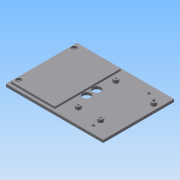
# Autodesk Inventor part: base_plate_r2
Saved by Autodesk Inventor 2014 (Build 180170000, 170)
## iProperties
Created: 2014-07-01
Part Number: base_plate_r2
Material: Generic
Document SubType Name: Modeling
Designer: Workstation
Density: 1 g/cm^3
Appearance: Default
Author: Workstation
Autodesk Inventor part; units mm, degrees
ref_plane "YZ Plane" through (0, 0, 0) normal (1, 0, 0) x (0, 1, 0)
ref_plane "XZ Plane" through (0, 0, 0) normal (0, 1, 0) x (-1, 0, 0)
ref_plane "XY Plane" through (0, 0, 0) normal (0, 0, 1) x (1, 0, 0)
sketch "Sketch1" plane through (0, 0, 0) normal (0, 1, 0) x (-1, 0, 0)
  line L0 (-16.8496, 81.8638) -> (105.0704, 81.8638)
  line L1 (105.0704, 81.8638) -> (105.0704, -7.0362)
  line L2 (105.0704, -7.0362) -> (-16.8496, -7.0362)
  line L3 (-16.8496, -7.0362) -> (-16.8496, 81.8638)
  point P0 (0, 0)
  dimension "d0" = 121.92
  dimension "d1" = 88.9
  constraints: 8 end point, 2 parallel, 1 horizontal, 1 perpendicular
  measures "d0" distance of L1.end L2.end
  measures "d1" distance of L0.end L1.end
extrude "Extrusion1" add sketch "Sketch1" along normal blind 3.429
sketch "Sketch2" plane through (0, 3.429, 0) normal (0, 1, 0) x (1, 0, 0)
  line L0 (-105.0704, -81.8638) -> (16.8496, -81.8638) projected
  line L1 (16.8496, 7.0362) -> (-105.0704, 7.0362) projected
  line L2 (-105.0704, 7.0362) -> (-105.0704, -81.8638) projected
  circle A0 centre (-98.7204, -2.6158) radius 1.5875
  circle A1 centre (-98.7204, -72.2118) radius 1.5875
  circle A2 centre (-4.7404, -2.6158) radius 1.5875
  circle A3 centre (-4.7404, -72.2118) radius 1.5875
  point P0 (0, 0)
  dimension "d4" = 121.92
  dimension "d5" = 88.9
  dimension "d6" = 6.35
  dimension "d8" = 6.35
  dimension "d12" = 3.175
  dimension "d13" = 3.175
  dimension "d15" = 3.175
  dimension "d18" = 93.98
  dimension "d20" = 69.596
  dimension "d21" = 9.652
  dimension "d22" = 9.652
  dimension "d23" = 3.175
  dimension "d64" = 9.652
  dimension "d65" = 9.652
  constraints: 4 centre point, 4 coincident
  measures "d4" distance of L0.start L0.end
  measures "d5" distance of L0.end L1.start
  measures "d6" distance from line of point (-98.72, -2.616) L2
  measures "d8" distance from line of point (-98.72, -72.212) L2
  measures "d12" diameter of A0
  measures "d13" diameter of A1
  measures "d15" diameter of A2
  measures "d18" distance of A0.centre A2.centre
  measures "d20" distance of A1.centre A0.centre
  measures "d21" distance from line of L1 A0.centre
  measures "d22" distance from line of L0 A1.centre
  measures "d23" diameter of A3
  measures "d64" distance from line of L1 A2.centre
  measures "d65" distance from line of L0 A3.centre
extrude "Extrusion3" cut sketch "Sketch2" against normal through all
sketch "Sketch4" plane through (0, 3.429, 0) normal (0, 1, 0) x (1, 0, 0)
  circle A0 centre (-98.7204, -2.6158) radius 1.5875 projected
  circle A1 centre (-98.7204, -72.2118) radius 1.5875 projected
  line L0 (16.8496, 7.0362) -> (-105.0704, 7.0362) projected
  line L1 (-105.0704, 7.0362) -> (-105.0704, -81.8638) projected
  line L2 (-101.8954, -78.6888) -> (-47.0314, -78.6888)
  line L3 (-47.0314, -78.6888) -> (-47.0314, 3.8612)
  line L4 (-47.0314, 3.8612) -> (-101.8954, 3.8612)
  line L5 (-101.8954, 3.8612) -> (-101.8954, -78.6888)
  circle A2 centre (-98.7204, -2.6158) radius 3.175
  circle A3 centre (-98.7204, -72.2118) radius 3.175
  point P0 (0, 0)
  dimension "d26" = 54.864
  dimension "d27" = 82.55
  dimension "d28" = 3.175
  dimension "d29" = 3.175
  dimension "d38" = 3.175
  constraints: 8 end point, 2 centre point, 2 coincident, 2 parallel, 2 perpendicular, 2 tangent
  measures "d26" distance of L2.start L2.end
  measures "d27" distance of L2.end L3.end
  measures "d28" distance between parallel lines of L4 L0
  measures "d29" distance between parallel lines of L5 L1
  measures "d38" distance from line of L5 A2.centre
extrude "Extrusion4" add sketch "Sketch4" along normal blind 2.54 contours L5 L4 L3 L2
sketch "Sketch5" plane through (0, 3.429, 0) normal (0, 1, 0) x (1, 0, 0)
  line L0 (-47.0314, 3.8612) -> (-47.0314, -78.6888) projected
  line L1 (-47.0314, -37.4138) -> (-47.0314, -31.0638)
  line L2 (-47.0314, -31.0638) -> (-47.0314, -43.7638)
  line L3 (-47.0314, -43.7638) -> (-41.9514, -43.7638)
  circle A0 centre (-41.9514, -43.7638) radius 5.08
  circle A1 centre (-41.9514, -31.0638) radius 5.08
  point P0 (0, 0)
  dimension "d35" = 6.35
  dimension "d36" = 12.7
  dimension "d37" = 5.08
  constraints: 6 end point, 2 horizontal alignment, 2 point on line, 1 coincident, 1 midpoint, 1 perpendicular, 4 other
  measures "d35" distance of L1.start L1.end
  measures "d36" distance of L1.end L2.end
  measures "d37" distance of L2.end L3.end
extrude "Extrusion5" cut sketch "Sketch5" against normal through all
sketch "Sketch6" plane through (0, 3.429, 0) normal (0, 1, 0) x (1, 0, 0)
  line L0 (-47.0314, -31.0638) -> (-47.0314, -43.7638) projected
  line L1 (-105.0704, 7.0362) -> (-105.0704, -81.8638) projected
  line L2 (-47.0314, -37.4138) -> (-40.6814, -37.4138)
  line L3 (-40.6814, -37.4138) -> (-40.6814, -65.3538)
  line L4 (-40.6814, -65.3538) -> (-40.6814, 3.1754)
  line L5 (-40.6814, 3.1754) -> (12.6586, 3.1754)
  line L6 (12.6586, 3.1754) -> (12.6586, -65.3538)
  line L7 (12.6586, -65.3538) -> (-40.6814, -65.3538)
  line L8 (-40.6814, -65.3538) -> (-40.6814, -63.0678)
  line L9 (-40.6814, -63.0678) -> (12.6586, -63.0678)
  line L10 (-40.6814, -63.0678) -> (-33.0614, -63.0678)
  line L11 (-33.0614, -63.0678) -> (-5.1214, -63.0678)
  circle A0 centre (-33.0614, -63.0678) radius 3.175
  circle A1 centre (-5.1214, -63.0678) radius 3.175
  line L12 (-40.6814, 3.1754) -> (-38.3954, 3.1754)
  line L13 (-38.3954, 3.1754) -> (-38.3954, -65.3538)
  line L14 (-38.3954, 3.1754) -> (-38.3954, -10.6168)
  circle A2 centre (-38.3954, -10.6168) radius 3.175
  line L15 (10.3726, 3.1754) -> (10.3726, -11.7598)
  circle A3 centre (10.3726, -11.7598) radius 3.175
  point P0 (0, 0)
  dimension "d39" = 6.35
  dimension "d40" = 27.94
  dimension "d41" = 68.5292
  dimension "d42" = 53.34
  dimension "d43" = 2.286
  dimension "d44" = 7.62
  dimension "d45" = 27.94
  dimension "d46" = 6.35
  dimension "d47" = 6.35
  dimension "d48" = 2.286
  dimension "d49" = 13.7922
  dimension "d50" = 6.35
  dimension "d51" = 14.9352
  dimension "d52" = 2.286
  dimension "d53" = 6.35
  constraints: 28 end point, 9 point on line, 6 perpendicular, 4 centre point, 4 coincident, 2 parallel, 1 midpoint
  measures "d39" distance of L2.start L2.end
  measures "d40" distance of L2.end L3.end
  measures "d41" distance of L3.end L4.end
  measures "d42" distance of L4.end L5.end
  measures "d43" distance of L3.end L8.end
  measures "d44" distance of L8.end L10.end
  measures "d45" distance of L10.end L11.end
  measures "d46" diameter of A0
  measures "d47" diameter of A1
  measures "d48" distance of L4.end L12.end
  measures "d49" distance of L12.end L14.end
  measures "d50" diameter of A2
  measures "d51" distance of L15.start L15.end
  measures "d52" distance between parallel lines of L6 L15
  measures "d53" diameter of A3
extrude "Extrusion6" add sketch "Sketch6" along normal blind 3.81 contours A2 L4 | L4 A2 L13 | L13 A2 | A0 L9 | L9 A0 L7 | L7 A0 | A1 L9 | L9 A1 L7 | L7 A1 | A3 L6 | A3 L6
sketch "Sketch7" plane through (-38.3954, 7.239, 10.6168) normal (0, 1, 0) x (1, 0, 0)
  circle A0 centre (48.768, -1.143) radius 3.175 projected
  circle A1 centre (33.274, -52.451) radius 3.175 projected
  circle A2 centre (5.334, -52.451) radius 3.175 projected
  circle A3 centre (48.768, -1.143) radius 1.27
  point P0 (38.3954, 10.6168)
  dimension "d56" = 2.54
  constraints: 1 centre point, 1 coincident
  measures "d56" diameter of A3
extrude "Extrusion7" add sketch "Sketch7" along normal blind 2.54 contours A3
sketch "Sketch8" plane through (-38.3954, 7.239, 10.6168) normal (0, 1, 0) x (1, 0, 0)
  circle A0 centre (0, 0) radius 3.175 projected
  circle A1 centre (5.334, -52.451) radius 3.175 projected
  circle A2 centre (33.274, -52.451) radius 3.175 projected
  circle A3 centre (0, 0) radius 1.0605
  circle A4 centre (5.334, -52.451) radius 1.0605
  circle A5 centre (33.274, -52.451) radius 1.0604
  point P0 (38.3954, 10.6168)
  dimension "d59" = 2.1209
  dimension "d60" = 2.1209
  dimension "d61" = 2.1209
  constraints: 3 centre point, 3 coincident
  measures "d59" diameter of A3
  measures "d60" diameter of A4
  measures "d61" diameter of A5
extrude "Extrusion8" cut sketch "Sketch8" against normal through all contours A3 | A4 | A5
body "Solid1"
